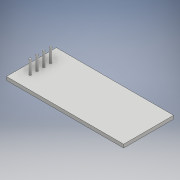
# Autodesk Inventor part: Zijplaat 3
Saved by Autodesk Inventor 2018.3 (Build 223284000, 284)
## iProperties
Created: 2020-11-10
Part Number: Zijplaat 3
Material: Generic
Document SubType Name: Modeling
Designer: daanv
Density: 1 g/cm^3
Appearance: Default
Author: daanv
Autodesk Inventor part; units mm, degrees
ref_plane "YZ Plane" through (0, 0, 0) normal (1, 0, 0) x (0, 1, 0)
ref_plane "XZ Plane" through (0, 0, 0) normal (0, 1, 0) x (-1, 0, 0)
ref_plane "XY Plane" through (0, 0, 0) normal (0, 0, 1) x (1, 0, 0)
sketch "Sketch1" plane through (0, 0, 0) normal (0, 0, 1) x (1, 0, 0)
  line L0 (0, 0) -> (0, 14.7)
  line L1 (0, 14.7) -> (34.5, 14.7)
  line L2 (34.5, 14.7) -> (34.5, 0)
  line L3 (34.5, 0) -> (0, 0)
  dimension "d0" = 14.7
  dimension "d1" = 34.5
  constraints: 8 end point, 3 perpendicular, 1 vertical
  measures "d0" distance of L0.start L0.end
  measures "d1" distance of L0.end L1.end
extrude "Extrusion1" add sketch "Sketch1" along normal blind 1
sketch "Sketch3" plane through (0, 0, 1) normal (0, 0, 1) x (1, 0, 0)
  circle A0 centre (3, 4) radius 0.325
  circle A1 centre (3, 6) radius 0.325
  circle A2 centre (3, 8) radius 0.325
  circle A3 centre (3, 10) radius 0.325
  dimension "d9" = 0.65
  dimension "d10" = 0.65
  dimension "d11" = 0.65
  dimension "d12" = 0.65
  constraints: 4 centre point, 4 coincident
  measures "d9" diameter of A0
  measures "d10" diameter of A1
  measures "d11" diameter of A2
  measures "d12" diameter of A3
extrude "Extrusion3" add sketch "Sketch3" along normal blind 4
body "Solid1"
